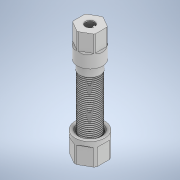
# Autodesk Inventor part: Shift Knob Adapter
Saved by Autodesk Inventor 2021 (Build 250183000, 183)
## iProperties
Created: 2022-01-31
Part Number: Shift Knob Adapter
Material: Generic
Document SubType Name: Modeling
Designer: Andrew
Density: 1 g/cm^3
Appearance: Default
Author: Andrew
Autodesk Inventor part; units mm, degrees
ref_plane "YZ Plane" through (0, 0, 0) normal (1, 0, 0) x (0, 1, 0)
ref_plane "XZ Plane" through (0, 0, 0) normal (0, 1, 0) x (-1, 0, 0)
ref_plane "XY Plane" through (0, 0, 0) normal (0, 0, 1) x (1, 0, 0)
sketch "Adapter Screw" plane through (0, 0, 0) normal (0, 0, 1) x (1, 0, 0)
  line L0 (7.75, 0) -> (7.75, 65.5)
  line L1 (7.75, 65.5) -> (9.15, 66.9)
  line L2 (9.15, 66.9) -> (9.15, 75)
  line L3 (9.15, 75) -> (11.25, 75)
  line L4 (11.25, 75) -> (11.25, 102)
  line L5 (6.05, 101) -> (6.05, 0)
  line L6 (6.05, 0) -> (7.75, 0)
  line L7 (7.75, 0) -> (7.75, -1.25)
  line L8 (8.75, -0.5) -> (7.75, 0)
  line L9 (8.75, -0.5) -> (8.75, -0.75)
  line L10 (8.75, -0.75) -> (7.75, -1.25)
  line L11 (7.75, -0.625) -> (8.75, -0.625) construction
  line L12 (11.25, 102) -> (4.2, 102)
  line L13 (4.2, 102) -> (4.2, 101)
  line L14 (4.2, 101) -> (6.05, 101)
  line L15 (0, -21.9) -> (0, 122.65) projected
  line L16 (8.75, -0.5) -> (8.75, 66.5)
  line L17 (4.2, 101) -> (5.45, 73)
  line L18 (5.45, 73) -> (6.05, 73)
  line L19 (10, 102) -> (10, 87)
  line L20 (10, 87) -> (11.25, 85.75)
  line L21 (8.75, 3) -> (7.75, 2)
  line L22 (5.45, 6) -> (6.05, 6) construction
  line L23 (6.75, 8) -> (7.75, 8) construction
  line L24 (0, 0) -> (0, 15)
  line L25 (1, 0) -> (1, 14)
  arc A0 (1, 14) -> (0, 15) centre (0, 14) ccw
  line L26 (1, 0) -> (0, 0)
  line L27 (5.05, 102) -> (5.05, 101)
  line L28 (4.2, 102) -> (2.95, 102)
  line L29 (2.95, 102) -> (2.95, 97.3312)
  line L30 (2.95, 97.3312) -> (4.6464, 91)
  arc A1 (6.05, 7.5) -> (6.05, 4.5) centre (7.625, 6) ccw
  line L31 (4.2, 101) -> (2.95, 101)
  line L32 (7.75, 2) -> (6.9, 0)
  dimension "d0" = 75
  dimension "d3" = 7.75
  dimension "d4" = 8.75
  dimension "d5" = 0.25
  dimension "d6" = 1.25
  dimension "d7" = 9.15
  dimension "d8" = 6.05
  dimension "d9" = 11.25
  dimension "d12" = 27
  dimension "d28" = 0.6
  dimension "d29" = 1.85
  dimension "d30" = 28
  dimension "d35" = 10
  dimension "d42" = 45
  dimension "d43" = 15
  dimension "d72" = 45
  dimension "d74" = 9.5
  dimension "d75" = 45
  dimension "d84" = 8
  dimension "d88" = 1
  dimension "d89" = 15
  dimension "d95" = 1
  dimension "d97" = 10
  dimension "d100" = 1
  dimension "d101" = 15
  dimension "d102" = 3.1
  dimension "d103" = 95
  dimension "d104" = 3
  dimension "d105" = 0.6
  dimension "d106" = 2
  constraints: 65 end point, 18 point on line, 10 perpendicular, 6 vertical, 5 point on circle, 4 horizontal, 3 midpoint, 2 centre point, 1 tangent
  measures "d0" distance between parallel lines of L6 L3
  measures "d3" distance from line of L24.start L7
  measures "d4" distance from line of L24.start L9
  measures "d5" distance of L8.start L9.end
  measures "d6" distance of L0.start L7.end
  measures "d7" distance from line of L24.start L2
  measures "d8" distance from line of L24.start L5
  measures "d9" distance from line of L24.start L4
  measures "d12" distance between parallel lines of L3 L12
  measures "d28" distance of L17.end L18.end
  measures "d29" distance of L5.start L13.end
  measures "d30" distance between parallel lines of L18 L14
  measures "d35" distance between parallel lines of L15 L19
  measures "d42" angle of L19 L20
  measures "d43" distance from line of L12 L19.end
  measures "d72" angle of L21 L16
  measures "d74" distance from line of L0.end L3
  measures "d75" angle of L0 L1
  measures "d84" distance between parallel lines of L6 L23
  measures "d88" distance of L25.start L24.start
  measures "d89" distance from line of L26 L24.end
  measures "d95" distance between parallel lines of L5 L27
  measures "d97" distance from line of L30.end L14
  measures "d100" distance between parallel lines of L12 L14
  measures "d101" angle of L29 L30
  measures "d102" distance between parallel lines of L5 L29
  measures "d103" distance between parallel lines of L14 L22
  measures "d104" distance of A1.end A1.start
  measures "d105" distance edge to line of A1 L5
  measures "d106" distance from line of L6 L21.end
sketch "Adapter Lock" plane through (0, 0, 0) normal (0, 0, 1) x (1, 0, 0)
  line L0 (8.375, -1.25) -> (9.375, -0.75)
  line L1 (9.375, -0.75) -> (9.375, -2)
  line L2 (9.375, -2) -> (8.375, -1.5)
  line L3 (8.375, -1.5) -> (8.375, -1.25)
  line L4 (8.375, -1.375) -> (9.375, -1.375) construction
  line L5 (7.75, -0.625) -> (8.75, -0.625) construction
  line L6 (9.375, 20) -> (13.25, 20)
  line L7 (13.25, 20) -> (13.25, 0)
  line L8 (13.25, 0) -> (9.375, 0)
  line L9 (9.375, 0) -> (9.375, 20)
  line L10 (9.15, 75) -> (11.25, 75) projected
  line L11 (12, 0) -> (12, 15)
  line L12 (12, 15) -> (13.25, 16.25)
  line L13 (9.375, 0) -> (8.375, 1)
  line L14 (8.375, 1) -> (8.375, 18)
  line L15 (8.375, 18) -> (9.375, 19)
  line L16 (0, -17.4) -> (0, 90.4) projected
  line L17 (9.375, 19) -> (10.375, 20)
  point P0 (0, 0)
  dimension "d44" = 0.25
  dimension "d45" = 1.25
  dimension "d46" = 1
  dimension "d47" = 8.375
  dimension "d48" = 0.75
  dimension "d49" = 13.25
  dimension "d50" = 55
  dimension "d51" = 20
  dimension "d52" = 12
  dimension "d53" = 15
  dimension "d54" = 45
  dimension "d55" = 45
  dimension "d56" = 45
  dimension "d107" = 1
  dimension "d108" = 1
  constraints: 30 end point, 4 parallel, 4 point on line, 2 collinear, 2 horizontal, 2 midpoint, 2 vertical, 1 perpendicular
  measures "d44" distance of L2.end L0.start
  measures "d45" distance of L0.end L1.end
  measures "d46" distance of L4.start L4.end
  measures "d47" distance from line of point (0, 0) L3
  measures "d48" distance between parallel lines of L4 L5
  measures "d49" distance from line of point (0, 0) L7
  measures "d50" distance between parallel lines of L6 L10
  measures "d51" distance of L6.end L7.end
  measures "d52" distance from line of point (0, 0) L11
  measures "d53" distance of L11.start L11.end
  measures "d54" angle of L7 L12
  measures "d55" angle of L9 L15
  measures "d56" angle of L9 L13
  measures "d107" distance from line of L15.end L6
  measures "d108" distance of L6.start L17.end
sketch "Sketch3" plane through (0, 0, 0) normal (0, 0, 1) x (1, 0, 0)
  point P0 (0, 0)
revolve "Revolution1" add sketch "Adapter Screw" angle 360 about axis through (0, -10, 0) along (0, 1, 0) contours L32 L6 L5 L14 L27 L12 L19 L20 L4 L3 L2 L1 L0 | A1 L5 | L20 L19 L12 L4 | L14 L13 L12 L27
coil "Coil1" sketch "Adapter Screw" operation add axis through (0, -10, 0) along (0, 1, 0) pitch 1.5 turns 50 hand right separate body contours L8 L9 L10 L7
revolve "Revolution2" cut sketch "Adapter Screw" angle 360 about axis through (0, -10, 0) along (0, 1, 0) keep common part bodies 2 contours L0 L1 L16 L21
combine bodies "Combine4" operation type add bodies to combine 1 2
chamfer "Chamfer1" distance 0.5 angle 45 1 edges at (-6.05, 0, 0)
extrude "Extrusion1" add sketch "Adapter Screw" along normal up to surface contours L18 L17 L14 L5 | L14 L13 L12 L27 round surface about axis through (0, 2.25, 0) along (0, -1, 0) radius 6.05 far side no bodies 1
extrude "Extrusion2" add sketch "Adapter Screw" against normal up to surface contours L18 L17 L14 L5 | L14 L13 L12 L27 round surface about axis through (0, 2.25, 0) along (0, -1, 0) radius 6.05 far side no bodies 1
extrude "Extrusion3" add sketch "Adapter Screw" along normal mid plane 20 separate body contours L20 L19 L12 L4
pattern_circular "Circular Pattern1" count 6 over 360 about axis through (0, -10, 0) along (0, 1, 0) bodies 3
combine bodies "Combine1" operation type subtract main body 1 bodies to subtract 3
revolve "Revolution3" add sketch "Adapter Lock" angle 360 about axis through (0, -10, 0) along (0, 1, 0) separate body contours L6 L7 L12 L11 L8 L9 L17 | L7 L8 L11 L12
extrude "Extrusion4" add sketch "Adapter Lock" along normal mid plane 20 separate body contours L7 L8 L11 L12
pattern_circular "Circular Pattern2" count 6 over 360 about axis through (0, -10, 0) along (0, 1, 0) bodies 5
combine bodies "Combine2" operation type subtract main body 4 bodies to subtract 5
coil "Coil2" sketch "Adapter Lock" operation add axis through (0, -10, 0) along (0, 1, 0) pitch 1.5 turns 50 hand right separate body contours L0 L1 L2 L3
revolve "Revolution4" cut sketch "Adapter Lock" angle 360 about axis through (0, -10, 0) along (0, 1, 0) keep common part bodies 6 contours L9 L13 L14 L15
combine bodies "Combine3" operation type add bodies to combine 4 6
extrude "Extrusion5" add sketch "Adapter Screw" along normal mid plane 20 separate body contours L15 A0 L25 L26
mirror "Mirror1" about plane through (0, 0, 0) normal (1, 0, 0) bodies 7
pattern_circular "Circular Pattern3" count 4 over 360 about axis through (0, -10, 0) along (0, 1, 0) bodies 7
combine bodies "Combine5" operation type subtract main body 1 bodies to subtract 7
extrude "Extrusion6" add sketch "Adapter Screw" along normal mid plane 2 contours L30 L29 L31 L17 | L31 L29 L28 L13 bodies 1
equation "\"d44\" = d5"
equation "\"d45\" = d6"
equation "\"d46\" = d4 - d3"
equation "\"d16\" = d0"
equation "\"d64\" = d0"
body "Solid1"
body "Solid4"
